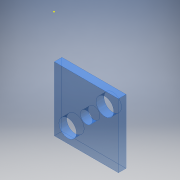
# Autodesk Inventor part: upperSeal
Saved by Autodesk Inventor 2016 (Build 200138000, 138)
## iProperties
Created: 2017-02-02
Part Number: upperSeal
Material: Water
Document SubType Name: Modeling
Designer: Teta
Density: 0.9983 g/cm^3
Appearance: Tropical Blue
Author: Teta
Autodesk Inventor part; units mm, degrees
ref_plane "YZ Plane" through (0, 0, 0) normal (1, 0, 0) x (0, 1, 0)
ref_plane "XZ Plane" through (0, 0, 0) normal (0, 1, 0) x (-1, 0, 0)
ref_plane "XY Plane" through (0, 0, 0) normal (0, 0, 1) x (1, 0, 0)
sketch "Sketch1" plane through (0, 0, 0) normal (0, 1, 0) x (-1, 0, 0)
  circle A0 centre (-20.0808, -22.2584) radius 3.45
  circle A1 centre (-5.4083, -36.9307) radius 3.45
  line L0 (-25.35, -17) -> (-25.35, -23.6)
  line L1 (-25.35, -23.6) -> (-25.35, -35.6)
  line L2 (-25.35, -35.6) -> (-25.35, -42.2)
  line L3 (-25.35, -42.2) -> (-0.15, -42.2)
  line L4 (-0.15, -42.2) -> (-0.15, -35.6)
  line L5 (-0.15, -35.6) -> (-0.15, -23.6)
  line L6 (-0.15, -23.6) -> (-0.15, -17)
  line L7 (-25.35, -42.2) -> (-0.15, -42.2)
  line L8 (-0.15, -42.2) -> (-0.15, -17)
  line L9 (-0.15, -17) -> (-25.35, -17)
  line L10 (-25.35, -17) -> (-25.35, -42.2)
  circle A2 centre (-12.75, -29.6) radius 2.075
  point P0 (0, 0)
  point P1 (0, 0)
  dimension "d0" = 25.2
  dimension "d1" = 4.15
  constraints: 22 end point, 3 centre point, 2 parallel, 1 horizontal, 1 perpendicular
  measures "d0" distance of L6.end L7.end
  measures "d1" diameter of A2
extrude "Extrusion1" add sketch "Sketch1" along normal blind 3
sketch "Sketch2" plane through (0, 0, 0) normal (0, -1, 0) x (1, 0, 0)
  point P0 (0, 0)
sketch "Sketch3" plane through (0, 0, 0) normal (0, -1, 0) x (1, 0, 0)
  circle A0 centre (12.75, -29.6) radius 2.075 projected
  circle A1 centre (12.75, -29.6) radius 2.15
  point P0 (0, 0)
  dimension "d4" = 4.3
  constraints: 1 centre point, 1 coincident
  measures "d4" diameter of A1
extrude "Extrusion2" cut sketch "Sketch3" against normal blind 10
sketch "Sketch4" plane through (0, 0, 0) normal (0, -1, 0) x (1, 0, 0)
  circle A0 centre (12.75, -29.6) radius 2.15 projected
  circle A1 centre (12.75, -29.6) radius 2.35
  point P0 (0, 0)
  dimension "d7" = 4.7
  constraints: 1 centre point, 1 coincident
  measures "d7" diameter of A1
extrude "Extrusion3" cut sketch "Sketch4" against normal blind 10
body "Solid1"
